Autodesk Inventor part; units mm, degrees
(part 2 of 3)
  circle A482 centre (-130.67, 0.7875) radius 0.851
  circle A483 centre (-28.5938, 38.8875) radius 1.994
  circle A484 centre (-33.6737, 38.8875) radius 0.851
  circle A485 centre (-23.5138, 38.8875) radius 0.851
  circle A486 centre (-19.0688, 19.8375) radius 1.994
  circle A487 centre (-24.1488, 19.8375) radius 0.851
  circle A488 centre (-13.9888, 19.8375) radius 0.851
  circle A489 centre (-14.3063, 0.7875) radius 1.994
  circle A490 centre (-19.3863, 0.7875) radius 0.851
  circle A491 centre (-9.2263, 0.7875) radius 0.851
  circle A492 centre (-4.7812, -18.2625) radius 1.994
  circle A493 centre (-9.8613, -18.2625) radius 0.851
  circle A494 centre (0.2988, -18.2625) radius 0.851
  circle A495 centre (-21.45, -37.3125) radius 1.994
  circle A496 centre (-26.53, -37.3125) radius 0.851
  circle A497 centre (-16.37, -37.3125) radius 0.851
  circle A498 centre (-71.488, -30.3275) radius 1.524
  circle A499 centre (28.588, -30.3275) radius 1.524
  circle A500 centre (-71.488, -45.5675) radius 1.994
  circle A501 centre (28.588, -45.5675) radius 1.994
  circle A502 centre (-9.5437, 38.8875) radius 1.994
  circle A503 centre (-14.6237, 38.8875) radius 0.851
  circle A504 centre (-4.4638, 38.8875) radius 0.851
  circle A505 centre (-0.0187, 19.8375) radius 1.994
  circle A506 centre (-5.0987, 19.8375) radius 0.851
  circle A507 centre (5.0613, 19.8375) radius 0.851
  circle A508 centre (4.7438, 0.7875) radius 1.994
  circle A509 centre (-0.3363, 0.7875) radius 0.851
  circle A510 centre (9.8238, 0.7875) radius 0.851
  circle A511 centre (14.2688, -18.2625) radius 1.994
  circle A512 centre (9.1888, -18.2625) radius 0.851
  circle A513 centre (19.3487, -18.2625) radius 0.851
  circle A514 centre (-130.9875, -18.2625) radius 1.994
  circle A515 centre (-136.0675, -18.2625) radius 0.851
  circle A516 centre (-125.9075, -18.2625) radius 0.851
  circle A517 centre (-142.9255, -11.2775) radius 1.524
  circle A518 centre (-119.0495, -11.2775) radius 1.524
  circle A519 centre (-142.9255, -26.5175) radius 1.994
  circle A520 centre (-119.0495, -26.5175) radius 1.994
  circle A521 centre (9.5063, 38.8875) radius 1.994
  circle A522 centre (4.4262, 38.8875) radius 0.851
  circle A523 centre (14.5862, 38.8875) radius 0.851
  circle A524 centre (19.0312, 19.8375) radius 1.994
  circle A525 centre (13.9513, 19.8375) radius 0.851
  circle A526 centre (24.1113, 19.8375) radius 0.851
  circle A527 centre (23.7937, 0.7875) radius 1.994
  circle A528 centre (18.7138, 0.7875) radius 0.851
  circle A529 centre (28.8738, 0.7875) radius 0.851
  circle A530 centre (33.3188, -18.2625) radius 1.994
  circle A531 centre (28.2388, -18.2625) radius 0.851
  circle A532 centre (38.3987, -18.2625) radius 0.851
  circle A533 centre (28.5562, 38.8875) radius 1.994
  circle A534 centre (23.4763, 38.8875) radius 0.851
  circle A535 centre (33.6362, 38.8875) radius 0.851
  circle A536 centre (38.0812, 19.8375) radius 1.994
  circle A537 centre (33.0012, 19.8375) radius 0.851
  circle A538 centre (43.1613, 19.8375) radius 0.851
  circle A539 centre (42.8438, 0.7875) radius 1.994
  circle A540 centre (37.7638, 0.7875) radius 0.851
  circle A541 centre (47.9237, 0.7875) radius 0.851
  circle A542 centre (52.3688, -18.2625) radius 1.994
  circle A543 centre (47.2888, -18.2625) radius 0.851
  circle A544 centre (57.4488, -18.2625) radius 0.851
  circle A545 centre (-140.5125, -37.3125) radius 1.994
  circle A546 centre (-145.5925, -37.3125) radius 0.851
  circle A547 centre (-135.4325, -37.3125) radius 0.851
  circle A548 centre (47.6063, 38.8875) radius 1.994
  circle A549 centre (42.5263, 38.8875) radius 0.851
  circle A550 centre (52.6863, 38.8875) radius 0.851
  circle A551 centre (57.1313, 19.8375) radius 1.994
  circle A552 centre (52.0513, 19.8375) radius 0.851
  circle A553 centre (62.2113, 19.8375) radius 0.851
  circle A554 centre (61.8937, 0.7875) radius 1.994
  circle A555 centre (56.8137, 0.7875) radius 0.851
  circle A556 centre (66.9737, 0.7875) radius 0.851
  circle A557 centre (71.4188, -18.2625) radius 1.994
  circle A558 centre (66.3388, -18.2625) radius 0.851
  circle A559 centre (76.4988, -18.2625) radius 0.851
  circle A560 centre (47.6063, -37.3125) radius 1.994
  circle A561 centre (42.5263, -37.3125) radius 0.851
  circle A562 centre (52.6863, -37.3125) radius 0.851
  circle A563 centre (66.6562, 38.8875) radius 1.994
  circle A564 centre (61.5763, 38.8875) radius 0.851
  circle A565 centre (71.7362, 38.8875) radius 0.851
  circle A566 centre (76.1813, 19.8375) radius 1.994
  circle A567 centre (71.1012, 19.8375) radius 0.851
  circle A568 centre (81.2613, 19.8375) radius 0.851
  circle A569 centre (80.9437, 0.7875) radius 1.994
  circle A570 centre (75.8638, 0.7875) radius 0.851
  circle A571 centre (86.0238, 0.7875) radius 0.851
  circle A572 centre (97.6125, -18.2625) radius 1.994
  circle A573 centre (92.5325, -18.2625) radius 0.851
  circle A574 centre (102.6925, -18.2625) radius 0.851
  circle A575 centre (-123.8438, 38.8875) radius 1.994
  circle A576 centre (-128.9238, 38.8875) radius 0.851
  circle A577 centre (-118.7638, 38.8875) radius 0.851
  circle A578 centre (66.6562, -37.3125) radius 1.994
  circle A579 centre (61.5763, -37.3125) radius 0.851
  circle A580 centre (71.7362, -37.3125) radius 0.851
  circle A581 centre (85.7062, 38.8875) radius 1.994
  circle A582 centre (80.6262, 38.8875) radius 0.851
  circle A583 centre (90.7863, 38.8875) radius 0.851
  circle A584 centre (95.2313, 19.8375) radius 1.994
  circle A585 centre (90.1513, 19.8375) radius 0.851
  circle A586 centre (100.3113, 19.8375) radius 0.851
  circle A587 centre (111.9, 0.7875) radius 1.994
  circle A588 centre (106.82, 0.7875) radius 0.851
  circle A589 centre (116.98, 0.7875) radius 0.851
  circle A590 centre (99.962, 7.7725) radius 1.524
  circle A591 centre (123.838, 7.7725) radius 1.524
  circle A592 centre (99.962, -7.4675) radius 1.994
  circle A593 centre (123.838, -7.4675) radius 1.994
  circle A594 centre (123.8063, -18.2625) radius 1.994
  circle A595 centre (118.7262, -18.2625) radius 0.851
  circle A596 centre (128.8862, -18.2625) radius 0.851
  circle A597 centre (85.7062, -37.3125) radius 1.994
  circle A598 centre (80.6262, -37.3125) radius 0.851
  circle A599 centre (90.7863, -37.3125) radius 0.851
  circle A600 centre (114.2813, 38.8875) radius 1.994
  circle A601 centre (109.2013, 38.8875) radius 0.851
  circle A602 centre (119.3613, 38.8875) radius 0.851
  circle A603 centre (102.3432, 45.8725) radius 1.524
  circle A604 centre (126.2193, 45.8725) radius 1.524
  circle A605 centre (102.3432, 30.6325) radius 1.994
  circle A606 centre (126.2193, 30.6325) radius 1.994
  circle A607 centre (119.0438, 19.8375) radius 1.994
  circle A608 centre (113.9638, 19.8375) radius 0.851
  circle A609 centre (124.1238, 19.8375) radius 0.851
  circle A610 centre (142.8562, 0.7875) radius 1.994
  circle A611 centre (137.7763, 0.7875) radius 0.851
  circle A612 centre (147.9363, 0.7875) radius 0.851
  circle A613 centre (142.8562, -18.2625) radius 1.994
  circle A614 centre (137.7763, -18.2625) radius 0.851
  circle A615 centre (147.9363, -18.2625) radius 0.851
  circle A616 centre (-114.3187, 19.8375) radius 1.994
  circle A617 centre (-119.3988, 19.8375) radius 0.851
  circle A618 centre (-109.2388, 19.8375) radius 0.851
  circle A619 centre (123.8063, -37.3125) radius 1.994
  circle A620 centre (118.7262, -37.3125) radius 0.851
  circle A621 centre (128.8862, -37.3125) radius 0.851
  circle A622 centre (142.8562, 38.8875) radius 1.994
  circle A623 centre (137.7763, 38.8875) radius 0.851
  circle A624 centre (147.9363, 38.8875) radius 0.851
  circle A625 centre (142.8562, 19.8375) radius 1.994
  circle A626 centre (137.7763, 19.8375) radius 0.851
  circle A627 centre (147.9363, 19.8375) radius 0.851
  circle A628 centre (104.7563, -37.3125) radius 1.994
  circle A629 centre (99.6762, -37.3125) radius 0.851
  circle A630 centre (109.8363, -37.3125) radius 0.851
  circle A631 centre (142.8562, -37.3125) radius 1.994
  circle A632 centre (137.7763, -37.3125) radius 0.851
  circle A633 centre (147.9363, -37.3125) radius 0.851
  circle A634 centre (-109.5563, 0.7875) radius 1.994
  circle A635 centre (-114.6363, 0.7875) radius 0.851
  circle A636 centre (-104.4763, 0.7875) radius 0.851
  circle A637 centre (-100.0312, -18.2625) radius 1.994
  circle A638 centre (-105.1112, -18.2625) radius 0.851
  circle A639 centre (-94.9513, -18.2625) radius 0.851
  line L281 (-145.2377, 58) -> (-145.2377, 70.7)
  line L282 (-153.25, 48.1608) -> (-159.6, 48.1608)
  line L283 (144.4828, -58) -> (144.4828, -70.7)
  line L284 (153.25, -45.7916) -> (159.6, -45.7916)
  line L285 (-159.6, 70.7) -> (159.6, 70.7)
  line L286 (159.6, 70.7) -> (159.6, -70.7)
  line L287 (159.6, -70.7) -> (-159.6, -70.7)
  line L288 (-159.6, -70.7) -> (-159.6, 70.7)
  line L289 (-149.6121, 31.8644) -> (-136.1755, 31.8644)
  line L290 (-135.8706, 32.1692) -> (-135.8706, 45.6058)
  line L291 (-136.1755, 45.9106) -> (-149.6121, 45.9106)
  line L292 (-149.9169, 45.6058) -> (-149.9169, 32.1692)
  line L293 (-149.9169, 31.8644) -> (-135.8706, 45.9106) construction
  line L294 (-135.8706, 31.8644) -> (-149.9169, 45.9106) construction
  arc A640 (-149.6121, 45.9106) -> (-149.9169, 45.6058) centre (-149.6121, 45.6058) ccw
  arc A641 (-135.8706, 45.6058) -> (-136.1755, 45.9106) centre (-136.1755, 45.6058) ccw
  arc A642 (-136.1755, 31.8644) -> (-135.8706, 32.1692) centre (-136.1755, 32.1692) ccw
  arc A643 (-149.9169, 32.1692) -> (-149.6121, 31.8644) centre (-149.6121, 32.1692) ccw
  line L295 (-130.562, 31.8644) -> (-117.1254, 31.8644)
  line L296 (-116.8206, 32.1692) -> (-116.8206, 45.6058)
  line L297 (-117.1254, 45.9106) -> (-130.562, 45.9106)
  line L298 (-130.8668, 45.6058) -> (-130.8668, 32.1692)
  line L299 (-130.8668, 31.8644) -> (-116.8206, 45.9106) construction
  line L300 (-116.8206, 31.8644) -> (-130.8668, 45.9106) construction
  arc A644 (-130.562, 45.9106) -> (-130.8668, 45.6058) centre (-130.562, 45.6058) ccw
  arc A645 (-116.8206, 45.6058) -> (-117.1254, 45.9106) centre (-117.1254, 45.6058) ccw
  arc A646 (-117.1254, 31.8644) -> (-116.8206, 32.1692) centre (-117.1254, 32.1692) ccw
  arc A647 (-130.8668, 32.1692) -> (-130.562, 31.8644) centre (-130.562, 32.1692) ccw
  line L301 (-111.5121, 31.8644) -> (-98.0754, 31.8644)
  line L302 (-97.7706, 32.1692) -> (-97.7706, 45.6058)
  line L303 (-98.0754, 45.9106) -> (-111.5121, 45.9106)
  line L304 (-111.8169, 45.6058) -> (-111.8169, 32.1692)
  line L305 (-111.8169, 31.8644) -> (-97.7706, 45.9106) construction
  line L306 (-97.7706, 31.8644) -> (-111.8169, 45.9106) construction
  arc A648 (-111.5121, 45.9106) -> (-111.8169, 45.6058) centre (-111.5121, 45.6058) ccw
  arc A649 (-97.7706, 45.6058) -> (-98.0754, 45.9106) centre (-98.0754, 45.6058) ccw
  arc A650 (-98.0754, 31.8644) -> (-97.7706, 32.1692) centre (-98.0754, 32.1692) ccw
  arc A651 (-111.8169, 32.1692) -> (-111.5121, 31.8644) centre (-111.512, 32.1692) ccw
  line L307 (-92.4621, 31.8644) -> (-79.0254, 31.8644)
  line L308 (-78.7206, 32.1692) -> (-78.7206, 45.6058)
  line L309 (-79.0254, 45.9106) -> (-92.4621, 45.9106)
  line L310 (-92.7669, 45.6058) -> (-92.7669, 32.1692)
  line L311 (-92.7669, 31.8644) -> (-78.7206, 45.9106) construction
  line L312 (-78.7206, 31.8644) -> (-92.7669, 45.9106) construction
  arc A652 (-92.4621, 45.9106) -> (-92.7669, 45.6058) centre (-92.4621, 45.6058) ccw
  arc A653 (-78.7206, 45.6058) -> (-79.0254, 45.9106) centre (-79.0255, 45.6058) ccw
  arc A654 (-79.0254, 31.8644) -> (-78.7206, 32.1692) centre (-79.0255, 32.1692) ccw
  arc A655 (-92.7669, 32.1692) -> (-92.4621, 31.8644) centre (-92.4621, 32.1692) ccw
  line L313 (-73.412, 31.8644) -> (-59.9754, 31.8644)
  line L314 (-59.6706, 32.1692) -> (-59.6706, 45.6058)
  line L315 (-59.9754, 45.9106) -> (-73.412, 45.9106)
  line L316 (-73.7168, 45.6058) -> (-73.7168, 32.1692)
  line L317 (-73.7168, 31.8644) -> (-59.6706, 45.9106) construction
  line L318 (-59.6706, 31.8644) -> (-73.7168, 45.9106) construction
  arc A656 (-73.412, 45.9106) -> (-73.7168, 45.6058) centre (-73.412, 45.6058) ccw
  arc A657 (-59.6706, 45.6058) -> (-59.9754, 45.9106) centre (-59.9754, 45.6058) ccw
  arc A658 (-59.9754, 31.8644) -> (-59.6706, 32.1692) centre (-59.9754, 32.1692) ccw
  arc A659 (-73.7168, 32.1692) -> (-73.412, 31.8644) centre (-73.412, 32.1692) ccw
  line L319 (-54.3621, 31.8644) -> (-40.9254, 31.8644)
  line L320 (-40.6206, 32.1692) -> (-40.6206, 45.6058)
  line L321 (-40.9254, 45.9106) -> (-54.3621, 45.9106)
  line L322 (-54.6668, 45.6058) -> (-54.6668, 32.1692)
  line L323 (-54.6668, 31.8644) -> (-40.6206, 45.9106) construction
  line L324 (-40.6206, 31.8644) -> (-54.6668, 45.9106) construction
  arc A660 (-54.3621, 45.9106) -> (-54.6668, 45.6058) centre (-54.3621, 45.6058) ccw
  arc A661 (-40.6206, 45.6058) -> (-40.9254, 45.9106) centre (-40.9254, 45.6058) ccw
  arc A662 (-40.9254, 31.8644) -> (-40.6206, 32.1692) centre (-40.9254, 32.1692) ccw
  arc A663 (-54.6668, 32.1692) -> (-54.3621, 31.8644) centre (-54.362, 32.1692) ccw
  line L325 (-35.312, 31.8644) -> (-21.8754, 31.8644)
  line L326 (-21.5706, 32.1692) -> (-21.5706, 45.6058)
  line L327 (-21.8754, 45.9106) -> (-35.312, 45.9106)
  line L328 (-35.6168, 45.6058) -> (-35.6168, 32.1692)
  line L329 (-35.6168, 31.8644) -> (-21.5706, 45.9106) construction
  line L330 (-21.5706, 31.8644) -> (-35.6168, 45.9106) construction
  arc A664 (-35.312, 45.9106) -> (-35.6168, 45.6058) centre (-35.312, 45.6058) ccw
  arc A665 (-21.5706, 45.6058) -> (-21.8754, 45.9106) centre (-21.8754, 45.6058) ccw
  arc A666 (-21.8754, 31.8644) -> (-21.5706, 32.1692) centre (-21.8754, 32.1692) ccw
  arc A667 (-35.6168, 32.1692) -> (-35.312, 31.8644) centre (-35.312, 32.1692) ccw
  line L331 (-16.262, 31.8644) -> (-2.8254, 31.8644)
  line L332 (-2.5206, 32.1692) -> (-2.5206, 45.6058)
  line L333 (-2.8254, 45.9106) -> (-16.262, 45.9106)
  line L334 (-16.5668, 45.6058) -> (-16.5668, 32.1692)
  line L335 (-16.5668, 31.8644) -> (-2.5206, 45.9106) construction
  line L336 (-2.5206, 31.8644) -> (-16.5668, 45.9106) construction
  arc A668 (-16.262, 45.9106) -> (-16.5668, 45.6058) centre (-16.262, 45.6058) ccw
  arc A669 (-2.5206, 45.6058) -> (-2.8254, 45.9106) centre (-2.8254, 45.6058) ccw
  arc A670 (-2.8254, 31.8644) -> (-2.5206, 32.1692) centre (-2.8254, 32.1692) ccw
  arc A671 (-16.5668, 32.1692) -> (-16.262, 31.8644) centre (-16.262, 32.1692) ccw
  line L337 (2.788, 31.8644) -> (16.2246, 31.8644)
  line L338 (16.5294, 32.1692) -> (16.5294, 45.6058)
  line L339 (16.2246, 45.9106) -> (2.788, 45.9106)
  line L340 (2.4832, 45.6058) -> (2.4832, 32.1692)
  line L341 (2.4832, 31.8644) -> (16.5294, 45.9106) construction
  line L342 (16.5294, 31.8644) -> (2.4832, 45.9106) construction
  arc A672 (2.788, 45.9106) -> (2.4832, 45.6058) centre (2.788, 45.6058) ccw
  arc A673 (16.5294, 45.6058) -> (16.2246, 45.9106) centre (16.2246, 45.6058) ccw
  arc A674 (16.2246, 31.8644) -> (16.5294, 32.1692) centre (16.2246, 32.1692) ccw
  arc A675 (2.4832, 32.1692) -> (2.788, 31.8644) centre (2.788, 32.1692) ccw
  line L343 (21.838, 31.8644) -> (35.2746, 31.8644)
  line L344 (35.5794, 32.1692) -> (35.5794, 45.6058)
  line L345 (35.2746, 45.9106) -> (21.838, 45.9106)
  line L346 (21.5332, 45.6058) -> (21.5332, 32.1692)
  line L347 (21.5332, 31.8644) -> (35.5794, 45.9106) construction
  line L348 (35.5794, 31.8644) -> (21.5332, 45.9106) construction
  arc A676 (21.838, 45.9106) -> (21.5332, 45.6058) centre (21.838, 45.6058) ccw
  arc A677 (35.5794, 45.6058) -> (35.2746, 45.9106) centre (35.2746, 45.6058) ccw
  arc A678 (35.2746, 31.8644) -> (35.5794, 32.1692) centre (35.2746, 32.1692) ccw
  arc A679 (21.5332, 32.1692) -> (21.838, 31.8644) centre (21.838, 32.1692) ccw
  line L349 (40.888, 31.8644) -> (54.3246, 31.8644)
  line L350 (54.6294, 32.1692) -> (54.6294, 45.6058)
  line L351 (54.3246, 45.9106) -> (40.888, 45.9106)
  line L352 (40.5832, 45.6058) -> (40.5832, 32.1692)
  line L353 (40.5832, 31.8644) -> (54.6294, 45.9106) construction
  line L354 (54.6294, 31.8644) -> (40.5832, 45.9106) construction
  arc A680 (40.888, 45.9106) -> (40.5832, 45.6058) centre (40.888, 45.6058) ccw
  arc A681 (54.6294, 45.6058) -> (54.3246, 45.9106) centre (54.3246, 45.6058) ccw
  arc A682 (54.3246, 31.8644) -> (54.6294, 32.1692) centre (54.3246, 32.1692) ccw
  arc A683 (40.5832, 32.1692) -> (40.888, 31.8644) centre (40.888, 32.1692) ccw
  line L355 (59.938, 31.8644) -> (73.3746, 31.8644)
  line L356 (73.6794, 32.1692) -> (73.6794, 45.6058)
  line L357 (73.3746, 45.9106) -> (59.938, 45.9106)
  line L358 (59.6332, 45.6058) -> (59.6332, 32.1692)
  line L359 (59.6332, 31.8644) -> (73.6794, 45.9106) construction
  line L360 (73.6794, 31.8644) -> (59.6332, 45.9106) construction
  arc A684 (59.938, 45.9106) -> (59.6332, 45.6058) centre (59.938, 45.6058) ccw
  arc A685 (73.6794, 45.6058) -> (73.3746, 45.9106) centre (73.3746, 45.6058) ccw
  arc A686 (73.3746, 31.8644) -> (73.6794, 32.1692) centre (73.3746, 32.1692) ccw
  arc A687 (59.6332, 32.1692) -> (59.938, 31.8644) centre (59.938, 32.1692) ccw
  line L361 (78.988, 31.8644) -> (92.4246, 31.8644)
  line L362 (92.7294, 32.1692) -> (92.7294, 45.6058)
  line L363 (92.4246, 45.9106) -> (78.988, 45.9106)
  line L364 (78.6832, 45.6058) -> (78.6832, 32.1692)
  line L365 (78.6832, 31.8644) -> (92.7294, 45.9106) construction
  line L366 (92.7294, 31.8644) -> (78.6832, 45.9106) construction
  arc A688 (78.988, 45.9106) -> (78.6832, 45.6058) centre (78.988, 45.6058) ccw
  arc A689 (92.7294, 45.6058) -> (92.4246, 45.9106) centre (92.4246, 45.6058) ccw
  arc A690 (92.4246, 31.8644) -> (92.7294, 32.1692) centre (92.4246, 32.1692) ccw
  arc A691 (78.6832, 32.1692) -> (78.988, 31.8644) centre (78.988, 32.1692) ccw
  line L367 (136.1379, 31.8644) -> (149.5746, 31.8644)
  line L368 (149.8794, 32.1692) -> (149.8794, 45.6058)
  line L369 (149.5746, 45.9106) -> (136.1379, 45.9106)
  line L370 (135.8332, 45.6058) -> (135.8332, 32.1692)
  line L371 (135.8332, 31.8644) -> (149.8794, 45.9106) construction
  line L372 (149.8794, 31.8644) -> (135.8332, 45.9106) construction
  arc A692 (136.1379, 45.9106) -> (135.8332, 45.6058) centre (136.1379, 45.6058) ccw
  arc A693 (149.8794, 45.6058) -> (149.5746, 45.9106) centre (149.5746, 45.6058) ccw
  arc A694 (149.5746, 31.8644) -> (149.8794, 32.1692) centre (149.5746, 32.1692) ccw
  arc A695 (135.8332, 32.1692) -> (136.1379, 31.8644) centre (136.138, 32.1692) ccw
  line L373 (-121.037, 12.8144) -> (-107.6004, 12.8144)
  line L374 (-107.2956, 13.1192) -> (-107.2956, 26.5558)
  line L375 (-107.6004, 26.8606) -> (-121.037, 26.8606)
  line L376 (-121.3418, 26.5558) -> (-121.3418, 13.1192)
  line L377 (-121.3418, 12.8144) -> (-107.2956, 26.8606) construction
  line L378 (-107.2956, 12.8144) -> (-121.3418, 26.8606) construction
  arc A696 (-121.037, 26.8606) -> (-121.3418, 26.5558) centre (-121.037, 26.5558) ccw
  arc A697 (-107.2956, 26.5558) -> (-107.6004, 26.8606) centre (-107.6004, 26.5558) ccw
  arc A698 (-107.6004, 12.8144) -> (-107.2956, 13.1192) centre (-107.6004, 13.1192) ccw
  arc A699 (-121.3418, 13.1192) -> (-121.037, 12.8144) centre (-121.037, 13.1192) ccw
  line L379 (-101.9871, 12.8144) -> (-88.5504, 12.8144)
  line L380 (-88.2456, 13.1192) -> (-88.2456, 26.5558)
  line L381 (-88.5504, 26.8606) -> (-101.9871, 26.8606)
  line L382 (-102.2918, 26.5558) -> (-102.2918, 13.1192)
  line L383 (-102.2918, 12.8144) -> (-88.2456, 26.8606) construction
  line L384 (-88.2456, 12.8144) -> (-102.2918, 26.8606) construction
  arc A700 (-101.9871, 26.8606) -> (-102.2918, 26.5558) centre (-101.9871, 26.5558) ccw
  arc A701 (-88.2456, 26.5558) -> (-88.5504, 26.8606) centre (-88.5504, 26.5558) ccw
  arc A702 (-88.5504, 12.8144) -> (-88.2456, 13.1192) centre (-88.5504, 13.1192) ccw
  arc A703 (-102.2918, 13.1192) -> (-101.9871, 12.8144) centre (-101.987, 13.1192) ccw
  line L385 (-82.937, 12.8144) -> (-69.5004, 12.8144)
  line L386 (-69.1956, 13.1192) -> (-69.1956, 26.5558)
  line L387 (-69.5004, 26.8606) -> (-82.937, 26.8606)
  line L388 (-83.2418, 26.5558) -> (-83.2418, 13.1192)
  line L389 (-83.2418, 12.8144) -> (-69.1956, 26.8606) construction
  line L390 (-69.1956, 12.8144) -> (-83.2418, 26.8606) construction
  arc A704 (-82.937, 26.8606) -> (-83.2418, 26.5558) centre (-82.937, 26.5558) ccw
  arc A705 (-69.1956, 26.5558) -> (-69.5004, 26.8606) centre (-69.5005, 26.5558) ccw
  arc A706 (-69.5004, 12.8144) -> (-69.1956, 13.1192) centre (-69.5005, 13.1192) ccw
  arc A707 (-83.2418, 13.1192) -> (-82.937, 12.8144) centre (-82.937, 13.1192) ccw
  line L391 (-63.887, 12.8144) -> (-50.4504, 12.8144)
  line L392 (-50.1456, 13.1192) -> (-50.1456, 26.5558)
  line L393 (-50.4504, 26.8606) -> (-63.887, 26.8606)
  line L394 (-64.1918, 26.5558) -> (-64.1918, 13.1192)
  line L395 (-64.1918, 12.8144) -> (-50.1456, 26.8606) construction
  line L396 (-50.1456, 12.8144) -> (-64.1918, 26.8606) construction
  arc A708 (-63.887, 26.8606) -> (-64.1918, 26.5558) centre (-63.887, 26.5558) ccw
  arc A709 (-50.1456, 26.5558) -> (-50.4504, 26.8606) centre (-50.4504, 26.5558) ccw
  arc A710 (-50.4504, 12.8144) -> (-50.1456, 13.1192) centre (-50.4504, 13.1192) ccw
  arc A711 (-64.1918, 13.1192) -> (-63.887, 12.8144) centre (-63.887, 13.1192) ccw
  line L397 (-44.837, 12.8144) -> (-31.4004, 12.8144)
  line L398 (-31.0956, 13.1192) -> (-31.0956, 26.5558)
  line L399 (-31.4004, 26.8606) -> (-44.837, 26.8606)
  line L400 (-45.1418, 26.5558) -> (-45.1418, 13.1192)
  line L401 (-45.1418, 12.8144) -> (-31.0956, 26.8606) construction
  line L402 (-31.0956, 12.8144) -> (-45.1418, 26.8606) construction
  arc A712 (-44.837, 26.8606) -> (-45.1418, 26.5558) centre (-44.837, 26.5558) ccw
  arc A713 (-31.0956, 26.5558) -> (-31.4004, 26.8606) centre (-31.4004, 26.5558) ccw
  arc A714 (-31.4004, 12.8144) -> (-31.0956, 13.1192) centre (-31.4004, 13.1192) ccw
  arc A715 (-45.1418, 13.1192) -> (-44.837, 12.8144) centre (-44.837, 13.1192) ccw
  line L403 (-25.787, 12.8144) -> (-12.3504, 12.8144)
  line L404 (-12.0456, 13.1192) -> (-12.0456, 26.5558)
  line L405 (-12.3504, 26.8606) -> (-25.787, 26.8606)
  line L406 (-26.0918, 26.5558) -> (-26.0918, 13.1192)
  line L407 (-26.0918, 12.8144) -> (-12.0456, 26.8606) construction
  line L408 (-12.0456, 12.8144) -> (-26.0918, 26.8606) construction
  arc A716 (-25.787, 26.8606) -> (-26.0918, 26.5558) centre (-25.787, 26.5558) ccw
  arc A717 (-12.0456, 26.5558) -> (-12.3504, 26.8606) centre (-12.3504, 26.5558) ccw
  arc A718 (-12.3504, 12.8144) -> (-12.0456, 13.1192) centre (-12.3504, 13.1192) ccw
  arc A719 (-26.0918, 13.1192) -> (-25.787, 12.8144) centre (-25.787, 13.1192) ccw
  line L409 (-6.737, 12.8144) -> (6.6996, 12.8144)
  line L410 (7.0044, 13.1192) -> (7.0044, 26.5558)
  line L411 (6.6996, 26.8606) -> (-6.737, 26.8606)
  line L412 (-7.0418, 26.5558) -> (-7.0418, 13.1192)
  line L413 (-7.0418, 12.8144) -> (7.0044, 26.8606) construction
  line L414 (7.0044, 12.8144) -> (-7.0418, 26.8606) construction
  arc A720 (-6.737, 26.8606) -> (-7.0418, 26.5558) centre (-6.737, 26.5558) ccw
  arc A721 (7.0044, 26.5558) -> (6.6996, 26.8606) centre (6.6996, 26.5558) ccw
  arc A722 (6.6996, 12.8144) -> (7.0044, 13.1192) centre (6.6996, 13.1192) ccw
  arc A723 (-7.0418, 13.1192) -> (-6.737, 12.8144) centre (-6.737, 13.1192) ccw
  line L415 (12.313, 12.8144) -> (25.7496, 12.8144)
  line L416 (26.0544, 13.1192) -> (26.0544, 26.5558)
  line L417 (25.7496, 26.8606) -> (12.313, 26.8606)
  line L418 (12.0082, 26.5558) -> (12.0082, 13.1192)
  line L419 (12.0082, 12.8144) -> (26.0544, 26.8606) construction
  line L420 (26.0544, 12.8144) -> (12.0082, 26.8606) construction
  arc A724 (12.313, 26.8606) -> (12.0082, 26.5558) centre (12.313, 26.5558) ccw
  arc A725 (26.0544, 26.5558) -> (25.7496, 26.8606) centre (25.7496, 26.5558) ccw
  arc A726 (25.7496, 12.8144) -> (26.0544, 13.1192) centre (25.7496, 13.1192) ccw
  arc A727 (12.0082, 13.1192) -> (12.313, 12.8144) centre (12.313, 13.1192) ccw
  line L421 (31.363, 12.8144) -> (44.7996, 12.8144)
  line L422 (45.1044, 13.1192) -> (45.1044, 26.5558)
  line L423 (44.7996, 26.8606) -> (31.363, 26.8606)
  line L424 (31.0582, 26.5558) -> (31.0582, 13.1192)
  line L425 (31.0582, 12.8144) -> (45.1044, 26.8606) construction
  line L426 (45.1044, 12.8144) -> (31.0582, 26.8606) construction
  arc A728 (31.363, 26.8606) -> (31.0582, 26.5558) centre (31.363, 26.5558) ccw
  arc A729 (45.1044, 26.5558) -> (44.7996, 26.8606) centre (44.7996, 26.5558) ccw
  arc A730 (44.7996, 12.8144) -> (45.1044, 13.1192) centre (44.7996, 13.1192) ccw
  arc A731 (31.0582, 13.1192) -> (31.363, 12.8144) centre (31.363, 13.1192) ccw
  line L427 (50.413, 12.8144) -> (63.8496, 12.8144)
  line L428 (64.1544, 13.1192) -> (64.1544, 26.5558)
  line L429 (63.8496, 26.8606) -> (50.413, 26.8606)
  line L430 (50.1082, 26.5558) -> (50.1082, 13.1192)
  line L431 (50.1082, 12.8144) -> (64.1544, 26.8606) construction
  line L432 (64.1544, 12.8144) -> (50.1082, 26.8606) construction
  arc A732 (50.413, 26.8606) -> (50.1082, 26.5558) centre (50.413, 26.5558) ccw
  arc A733 (64.1544, 26.5558) -> (63.8496, 26.8606) centre (63.8496, 26.5558) ccw
  arc A734 (63.8496, 12.8144) -> (64.1544, 13.1192) centre (63.8496, 13.1192) ccw
  arc A735 (50.1082, 13.1192) -> (50.413, 12.8144) centre (50.413, 13.1192) ccw
  line L433 (69.463, 12.8144) -> (82.8996, 12.8144)
  line L434 (83.2044, 13.1192) -> (83.2044, 26.5558)
  line L435 (82.8996, 26.8606) -> (69.463, 26.8606)
  line L436 (69.1582, 26.5558) -> (69.1582, 13.1192)
  line L437 (69.1582, 12.8144) -> (83.2044, 26.8606) construction
  line L438 (83.2044, 12.8144) -> (69.1582, 26.8606) construction
  arc A736 (69.463, 26.8606) -> (69.1582, 26.5558) centre (69.463, 26.5558) ccw
  arc A737 (83.2044, 26.5558) -> (82.8996, 26.8606) centre (82.8996, 26.5558) ccw
  arc A738 (82.8996, 12.8144) -> (83.2044, 13.1192) centre (82.8996, 13.1192) ccw
  arc A739 (69.1582, 13.1192) -> (69.463, 12.8144) centre (69.463, 13.1192) ccw
  line L439 (88.513, 12.8144) -> (101.9496, 12.8144)
  line L440 (102.2544, 13.1192) -> (102.2544, 26.5558)
  line L441 (101.9496, 26.8606) -> (88.513, 26.8606)
  line L442 (88.2082, 26.5558) -> (88.2082, 13.1192)
  line L443 (88.2082, 12.8144) -> (102.2544, 26.8606) construction
  line L444 (102.2544, 12.8144) -> (88.2082, 26.8606) construction
  arc A740 (88.513, 26.8606) -> (88.2082, 26.5558) centre (88.513, 26.5558) ccw
  arc A741 (102.2544, 26.5558) -> (101.9496, 26.8606) centre (101.9496, 26.5558) ccw
  arc A742 (101.9496, 12.8144) -> (102.2544, 13.1192) centre (101.9496, 13.1192) ccw
  arc A743 (88.2082, 13.1192) -> (88.513, 12.8144) centre (88.513, 13.1192) ccw
  line L445 (136.1379, 12.8144) -> (149.5746, 12.8144)
  line L446 (149.8794, 13.1192) -> (149.8794, 26.5558)
  line L447 (149.5746, 26.8606) -> (136.1379, 26.8606)
  line L448 (135.8332, 26.5558) -> (135.8332, 13.1192)
  line L449 (135.8332, 12.8144) -> (149.8794, 26.8606) construction
  line L450 (149.8794, 12.8144) -> (135.8332, 26.8606) construction
  arc A744 (136.1379, 26.8606) -> (135.8332, 26.5558) centre (136.1379, 26.5558) ccw
  arc A745 (149.8794, 26.5558) -> (149.5746, 26.8606) centre (149.5746, 26.5558) ccw
  arc A746 (149.5746, 12.8144) -> (149.8794, 13.1192) centre (149.5746, 13.1192) ccw
  arc A747 (135.8332, 13.1192) -> (136.1379, 12.8144) centre (136.138, 13.1192) ccw
  line L451 (-116.2746, -6.2356) -> (-102.8379, -6.2356)
  line L452 (-102.5331, -5.9308) -> (-102.5331, 7.5058)
  line L453 (-102.8379, 7.8106) -> (-116.2746, 7.8106)
  line L454 (-116.5794, 7.5058) -> (-116.5794, -5.9308)
  line L455 (-116.5794, -6.2356) -> (-102.5331, 7.8106) construction
  line L456 (-102.5331, -6.2356) -> (-116.5794, 7.8106) construction
  arc A748 (-116.2746, 7.8106) -> (-116.5794, 7.5058) centre (-116.2746, 7.5058) ccw
  arc A749 (-102.5331, 7.5058) -> (-102.8379, 7.8106) centre (-102.8379, 7.5058) ccw
  arc A750 (-102.8379, -6.2356) -> (-102.5331, -5.9308) centre (-102.8379, -5.9308) ccw
  arc A751 (-116.5794, -5.9308) -> (-116.2746, -6.2356) centre (-116.2745, -5.9308) ccw
  line L457 (-97.2245, -6.2356) -> (-83.7879, -6.2356)
  line L458 (-83.4831, -5.9308) -> (-83.4831, 7.5058)
  line L459 (-83.7879, 7.8106) -> (-97.2245, 7.8106)
  line L460 (-97.5293, 7.5058) -> (-97.5293, -5.9308)
  line L461 (-97.5293, -6.2356) -> (-83.4831, 7.8106) construction
  line L462 (-83.4831, -6.2356) -> (-97.5293, 7.8106) construction
  arc A752 (-97.2245, 7.8106) -> (-97.5293, 7.5058) centre (-97.2245, 7.5058) ccw
  arc A753 (-83.4831, 7.5058) -> (-83.7879, 7.8106) centre (-83.7879, 7.5058) ccw
  arc A754 (-83.7879, -6.2356) -> (-83.4831, -5.9308) centre (-83.7879, -5.9308) ccw
  arc A755 (-97.5293, -5.9308) -> (-97.2245, -6.2356) centre (-97.2245, -5.9308) ccw
  line L463 (-78.1745, -6.2356) -> (-64.7379, -6.2356)
  line L464 (-64.4331, -5.9308) -> (-64.4331, 7.5058)
  line L465 (-64.7379, 7.8106) -> (-78.1745, 7.8106)
  line L466 (-78.4793, 7.5058) -> (-78.4793, -5.9308)
  line L467 (-78.4793, -6.2356) -> (-64.4331, 7.8106) construction
  line L468 (-64.4331, -6.2356) -> (-78.4793, 7.8106) construction
  arc A756 (-78.1745, 7.8106) -> (-78.4793, 7.5058) centre (-78.1745, 7.5058) ccw
  arc A757 (-64.4331, 7.5058) -> (-64.7379, 7.8106) centre (-64.7379, 7.5058) ccw
  arc A758 (-64.7379, -6.2356) -> (-64.4331, -5.9308) centre (-64.7379, -5.9308) ccw
  arc A759 (-78.4793, -5.9308) -> (-78.1745, -6.2356) centre (-78.1745, -5.9308) ccw
  line L469 (-59.1245, -6.2356) -> (-45.6879, -6.2356)
  line L470 (-45.3831, -5.9308) -> (-45.3831, 7.5058)
  line L471 (-45.6879, 7.8106) -> (-59.1245, 7.8106)
  line L472 (-59.4293, 7.5058) -> (-59.4293, -5.9308)
  line L473 (-59.4293, -6.2356) -> (-45.3831, 7.8106) construction
  line L474 (-45.3831, -6.2356) -> (-59.4293, 7.8106) construction
  arc A760 (-59.1245, 7.8106) -> (-59.4293, 7.5058) centre (-59.1245, 7.5058) ccw
  arc A761 (-45.3831, 7.5058) -> (-45.6879, 7.8106) centre (-45.6879, 7.5058) ccw
  arc A762 (-45.6879, -6.2356) -> (-45.3831, -5.9308) centre (-45.6879, -5.9308) ccw
  arc A763 (-59.4293, -5.9308) -> (-59.1245, -6.2356) centre (-59.1245, -5.9308) ccw
  line L475 (-40.0745, -6.2356) -> (-26.6379, -6.2356)
  line L476 (-26.3331, -5.9308) -> (-26.3331, 7.5058)
  line L477 (-26.6379, 7.8106) -> (-40.0745, 7.8106)
  line L478 (-40.3793, 7.5058) -> (-40.3793, -5.9308)
  line L479 (-40.3793, -6.2356) -> (-26.3331, 7.8106) construction
  line L480 (-26.3331, -6.2356) -> (-40.3793, 7.8106) construction
  arc A764 (-40.0745, 7.8106) -> (-40.3793, 7.5058) centre (-40.0745, 7.5058) ccw
  arc A765 (-26.3331, 7.5058) -> (-26.6379, 7.8106) centre (-26.6379, 7.5058) ccw
  arc A766 (-26.6379, -6.2356) -> (-26.3331, -5.9308) centre (-26.6379, -5.9308) ccw
  arc A767 (-40.3793, -5.9308) -> (-40.0745, -6.2356) centre (-40.0745, -5.9308) ccw
  line L481 (-21.0245, -6.2356) -> (-7.5879, -6.2356)
  line L482 (-7.2831, -5.9308) -> (-7.2831, 7.5058)
  line L483 (-7.5879, 7.8106) -> (-21.0245, 7.8106)
  line L484 (-21.3293, 7.5058) -> (-21.3293, -5.9308)
  line L485 (-21.3293, -6.2356) -> (-7.2831, 7.8106) construction
  line L486 (-7.2831, -6.2356) -> (-21.3293, 7.8106) construction
  arc A768 (-21.0245, 7.8106) -> (-21.3293, 7.5058) centre (-21.0245, 7.5058) ccw
  arc A769 (-7.2831, 7.5058) -> (-7.5879, 7.8106) centre (-7.5879, 7.5058) ccw
  arc A770 (-7.5879, -6.2356) -> (-7.2831, -5.9308) centre (-7.5879, -5.9308) ccw
  arc A771 (-21.3293, -5.9308) -> (-21.0245, -6.2356) centre (-21.0245, -5.9308) ccw
  line L487 (-1.9745, -6.2356) -> (11.4621, -6.2356)
  line L488 (11.7669, -5.9308) -> (11.7669, 7.5058)
  line L489 (11.4621, 7.8106) -> (-1.9745, 7.8106)
  line L490 (-2.2793, 7.5058) -> (-2.2793, -5.9308)
  line L491 (-2.2793, -6.2356) -> (11.7669, 7.8106) construction
  line L492 (11.7669, -6.2356) -> (-2.2793, 7.8106) construction
  arc A772 (-1.9745, 7.8106) -> (-2.2793, 7.5058) centre (-1.9745, 7.5058) ccw
  arc A773 (11.7669, 7.5058) -> (11.4621, 7.8106) centre (11.4621, 7.5058) ccw
  arc A774 (11.4621, -6.2356) -> (11.7669, -5.9308) centre (11.4621, -5.9308) ccw
  arc A775 (-2.2793, -5.9308) -> (-1.9745, -6.2356) centre (-1.9745, -5.9308) ccw
  line L493 (17.0755, -6.2356) -> (30.5121, -6.2356)
  line L494 (30.8169, -5.9308) -> (30.8169, 7.5058)
  line L495 (30.5121, 7.8106) -> (17.0755, 7.8106)
  line L496 (16.7707, 7.5058) -> (16.7707, -5.9308)
  line L497 (16.7707, -6.2356) -> (30.8169, 7.8106) construction
  line L498 (30.8169, -6.2356) -> (16.7707, 7.8106) construction
  arc A776 (17.0755, 7.8106) -> (16.7707, 7.5058) centre (17.0755, 7.5058) ccw
  arc A777 (30.8169, 7.5058) -> (30.5121, 7.8106) centre (30.5121, 7.5058) ccw
  arc A778 (30.5121, -6.2356) -> (30.8169, -5.9308) centre (30.5121, -5.9308) ccw
  arc A779 (16.7707, -5.9308) -> (17.0755, -6.2356) centre (17.0755, -5.9308) ccw
  line L499 (36.1255, -6.2356) -> (49.5621, -6.2356)
  line L500 (49.8669, -5.9308) -> (49.8669, 7.5058)
  line L501 (49.5621, 7.8106) -> (36.1255, 7.8106)
  line L502 (35.8207, 7.5058) -> (35.8207, -5.9308)
  line L503 (35.8207, -6.2356) -> (49.8669, 7.8106) construction
  line L504 (49.8669, -6.2356) -> (35.8207, 7.8106) construction
  arc A780 (36.1255, 7.8106) -> (35.8207, 7.5058) centre (36.1255, 7.5058) ccw
  arc A781 (49.8669, 7.5058) -> (49.5621, 7.8106) centre (49.5621, 7.5058) ccw
  arc A782 (49.5621, -6.2356) -> (49.8669, -5.9308) centre (49.5621, -5.9308) ccw
  arc A783 (35.8207, -5.9308) -> (36.1255, -6.2356) centre (36.1255, -5.9308) ccw
  line L505 (55.1755, -6.2356) -> (68.6121, -6.2356)
  line L506 (68.9169, -5.9308) -> (68.9169, 7.5058)
  line L507 (68.6121, 7.8106) -> (55.1755, 7.8106)
  line L508 (54.8707, 7.5058) -> (54.8707, -5.9308)
  line L509 (54.8707, -6.2356) -> (68.9169, 7.8106) construction
  line L510 (68.9169, -6.2356) -> (54.8707, 7.8106) construction
  arc A784 (55.1755, 7.8106) -> (54.8707, 7.5058) centre (55.1755, 7.5058) ccw
  arc A785 (68.9169, 7.5058) -> (68.6121, 7.8106) centre (68.6121, 7.5058) ccw
  arc A786 (68.6121, -6.2356) -> (68.9169, -5.9308) centre (68.6121, -5.9308) ccw
  arc A787 (54.8707, -5.9308) -> (55.1755, -6.2356) centre (55.1755, -5.9308) ccw
  line L511 (74.2255, -6.2356) -> (87.6621, -6.2356)
  line L512 (87.9669, -5.9308) -> (87.9669, 7.5058)
  line L513 (87.6621, 7.8106) -> (74.2255, 7.8106)
  line L514 (73.9207, 7.5058) -> (73.9207, -5.9308)
  line L515 (73.9207, -6.2356) -> (87.9669, 7.8106) construction
  line L516 (87.9669, -6.2356) -> (73.9207, 7.8106) construction
  arc A788 (74.2255, 7.8106) -> (73.9207, 7.5058) centre (74.2255, 7.5058) ccw
  arc A789 (87.9669, 7.5058) -> (87.6621, 7.8106) centre (87.6621, 7.5058) ccw
  arc A790 (87.6621, -6.2356) -> (87.9669, -5.9308) centre (87.6621, -5.9308) ccw
  arc A791 (73.9207, -5.9308) -> (74.2255, -6.2356) centre (74.2255, -5.9308) ccw
  line L517 (136.1379, -6.2356) -> (149.5746, -6.2356)
  line L518 (149.8794, -5.9308) -> (149.8794, 7.5058)
  line L519 (149.5746, 7.8106) -> (136.1379, 7.8106)
  line L520 (135.8332, 7.5058) -> (135.8332, -5.9308)
  line L521 (135.8332, -6.2356) -> (149.8794, 7.8106) construction
  line L522 (149.8794, -6.2356) -> (135.8332, 7.8106) construction
  arc A792 (136.1379, 7.8106) -> (135.8332, 7.5058) centre (136.1379, 7.5058) ccw
  arc A793 (149.8794, 7.5058) -> (149.5746, 7.8106) centre (149.5746, 7.5058) ccw
  arc A794 (149.5746, -6.2356) -> (149.8794, -5.9308) centre (149.5746, -5.9308) ccw
  arc A795 (135.8332, -5.9308) -> (136.1379, -6.2356) centre (136.138, -5.9308) ccw
  line L523 (-106.7495, -25.2856) -> (-93.3129, -25.2856)
  line L524 (-93.0081, -24.9808) -> (-93.0081, -11.5442)
  line L525 (-93.3129, -11.2394) -> (-106.7495, -11.2394)
  line L526 (-107.0543, -11.5442) -> (-107.0543, -24.9808)
  line L527 (-107.0543, -25.2856) -> (-93.0081, -11.2394) construction
  line L528 (-93.0081, -25.2856) -> (-107.0543, -11.2394) construction
  arc A796 (-106.7495, -11.2394) -> (-107.0543, -11.5442) centre (-106.7495, -11.5442) ccw
  arc A797 (-93.0081, -11.5442) -> (-93.3129, -11.2394) centre (-93.3129, -11.5442) ccw
  arc A798 (-93.3129, -25.2856) -> (-93.0081, -24.9808) centre (-93.3129, -24.9808) ccw
  arc A799 (-107.0543, -24.9808) -> (-106.7495, -25.2856) centre (-106.7495, -24.9808) ccw
  line L529 (-87.6995, -25.2856) -> (-74.2629, -25.2856)
  line L530 (-73.9581, -24.9808) -> (-73.9581, -11.5442)
  line L531 (-74.2629, -11.2394) -> (-87.6995, -11.2394)
  line L532 (-88.0044, -11.5442) -> (-88.0044, -24.9808)
  line L533 (-88.0044, -25.2856) -> (-73.9581, -11.2394) construction
  line L534 (-73.9581, -25.2856) -> (-88.0044, -11.2394) construction
  arc A800 (-87.6995, -11.2394) -> (-88.0044, -11.5442) centre (-87.6995, -11.5442) ccw
  arc A801 (-73.9581, -11.5442) -> (-74.2629, -11.2394) centre (-74.2629, -11.5442) ccw
  arc A802 (-74.2629, -25.2856) -> (-73.9581, -24.9808) centre (-74.2629, -24.9808) ccw
  arc A803 (-88.0044, -24.9808) -> (-87.6995, -25.2856) centre (-87.6995, -24.9808) ccw
  line L535 (-68.7073, -25.2278) -> (-55.2707, -25.2278)
  line L536 (-54.9659, -24.923) -> (-54.9659, -11.4864)
  line L537 (-55.2707, -11.1816) -> (-68.7073, -11.1816)
  line L538 (-69.0121, -11.4864) -> (-69.0121, -24.923)
  line L539 (-69.0121, -25.2278) -> (-54.9659, -11.1816) construction
  line L540 (-54.9659, -25.2278) -> (-69.0121, -11.1816) construction
  arc A804 (-68.7073, -11.1816) -> (-69.0121, -11.4864) centre (-68.7073, -11.4864) ccw
  arc A805 (-54.9659, -11.4864) -> (-55.2707, -11.1816) centre (-55.2707, -11.4864) ccw
  arc A806 (-55.2707, -25.2278) -> (-54.9659, -24.923) centre (-55.2707, -24.923) ccw
  arc A807 (-69.0121, -24.923) -> (-68.7073, -25.2278) centre (-68.7073, -24.923) ccw
  line L541 (-49.5995, -25.2856) -> (-36.1629, -25.2856)
  line L542 (-35.8581, -24.9808) -> (-35.8581, -11.5442)
  line L543 (-36.1629, -11.2394) -> (-49.5995, -11.2394)
  line L544 (-49.9043, -11.5442) -> (-49.9043, -24.9808)
  line L545 (-49.9043, -25.2856) -> (-35.8581, -11.2394) construction
  line L546 (-35.8581, -25.2856) -> (-49.9043, -11.2394) construction
  arc A808 (-49.5995, -11.2394) -> (-49.9043, -11.5442) centre (-49.5995, -11.5442) ccw
  arc A809 (-35.8581, -11.5442) -> (-36.1629, -11.2394) centre (-36.1629, -11.5442) ccw
  arc A810 (-36.1629, -25.2856) -> (-35.8581, -24.9808) centre (-36.1629, -24.9808) ccw
  arc A811 (-49.9043, -24.9808) -> (-49.5995, -25.2856) centre (-49.5995, -24.9808) ccw
  line L547 (-30.5495, -25.2856) -> (-17.1129, -25.2856)
  line L548 (-16.8081, -24.9808) -> (-16.8081, -11.5442)
  line L549 (-17.1129, -11.2394) -> (-30.5495, -11.2394)
  line L550 (-30.8543, -11.5442) -> (-30.8543, -24.9808)
  line L551 (-30.8543, -25.2856) -> (-16.8081, -11.2394) construction
  line L552 (-16.8081, -25.2856) -> (-30.8543, -11.2394) construction
  arc A812 (-30.5495, -11.2394) -> (-30.8543, -11.5442) centre (-30.5495, -11.5442) ccw
  arc A813 (-16.8081, -11.5442) -> (-17.1129, -11.2394) centre (-17.1129, -11.5442) ccw
  arc A814 (-17.1129, -25.2856) -> (-16.8081, -24.9808) centre (-17.1129, -24.9808) ccw
  arc A815 (-30.8543, -24.9808) -> (-30.5495, -25.2856) centre (-30.5495, -24.9808) ccw
  line L553 (-11.4995, -25.2856) -> (1.9371, -25.2856)
  line L554 (2.2419, -24.9808) -> (2.2419, -11.5442)
  line L555 (1.9371, -11.2394) -> (-11.4995, -11.2394)
  line L556 (-11.8043, -11.5442) -> (-11.8043, -24.9808)
  line L557 (-11.8043, -25.2856) -> (2.2419, -11.2394) construction
  line L558 (2.2419, -25.2856) -> (-11.8043, -11.2394) construction
  arc A816 (-11.4995, -11.2394) -> (-11.8043, -11.5442) centre (-11.4995, -11.5442) ccw
  arc A817 (2.2419, -11.5442) -> (1.9371, -11.2394) centre (1.9371, -11.5442) ccw
  arc A818 (1.9371, -25.2856) -> (2.2419, -24.9808) centre (1.9371, -24.9808) ccw
  arc A819 (-11.8043, -24.9808) -> (-11.4995, -25.2856) centre (-11.4995, -24.9808) ccw
  line L559 (7.5505, -25.2856) -> (20.9871, -25.2856)
  line L560 (21.2919, -24.9808) -> (21.2919, -11.5442)
  line L561 (20.9871, -11.2394) -> (7.5505, -11.2394)
  line L562 (7.2457, -11.5442) -> (7.2457, -24.9808)
  line L563 (7.2457, -25.2856) -> (21.2919, -11.2394) construction
  line L564 (21.2919, -25.2856) -> (7.2457, -11.2394) construction
  arc A820 (7.5505, -11.2394) -> (7.2457, -11.5442) centre (7.5505, -11.5442) ccw
  arc A821 (21.2919, -11.5442) -> (20.9871, -11.2394) centre (20.9871, -11.5442) ccw
  arc A822 (20.9871, -25.2856) -> (21.2919, -24.9808) centre (20.9871, -24.9808) ccw
  arc A823 (7.2457, -24.9808) -> (7.5505, -25.2856) centre (7.5505, -24.9808) ccw
  line L565 (26.6005, -25.2856) -> (40.0371, -25.2856)
  line L566 (40.3419, -24.9808) -> (40.3419, -11.5442)
  line L567 (40.0371, -11.2394) -> (26.6005, -11.2394)
  line L568 (26.2957, -11.5442) -> (26.2957, -24.9808)
  line L569 (26.2957, -25.2856) -> (40.3419, -11.2394) construction
  line L570 (40.3419, -25.2856) -> (26.2957, -11.2394) construction
  arc A824 (26.6005, -11.2394) -> (26.2957, -11.5442) centre (26.6005, -11.5442) ccw
  arc A825 (40.3419, -11.5442) -> (40.0371, -11.2394) centre (40.0371, -11.5442) ccw
  arc A826 (40.0371, -25.2856) -> (40.3419, -24.9808) centre (40.0371, -24.9808) ccw
  arc A827 (26.2957, -24.9808) -> (26.6005, -25.2856) centre (26.6005, -24.9808) ccw
  line L571 (45.6505, -25.2856) -> (59.0871, -25.2856)
  line L572 (59.3919, -24.9808) -> (59.3919, -11.5442)
  line L573 (59.0871, -11.2394) -> (45.6505, -11.2394)
  line L574 (45.3457, -11.5442) -> (45.3457, -24.9808)
  line L575 (45.3457, -25.2856) -> (59.3919, -11.2394) construction
  line L576 (59.3919, -25.2856) -> (45.3457, -11.2394) construction
  arc A828 (45.6505, -11.2394) -> (45.3457, -11.5442) centre (45.6505, -11.5442) ccw
  arc A829 (59.3919, -11.5442) -> (59.0871, -11.2394) centre (59.0871, -11.5442) ccw
  arc A830 (59.0871, -25.2856) -> (59.3919, -24.9808) centre (59.0871, -24.9808) ccw
  arc A831 (45.3457, -24.9808) -> (45.6505, -25.2856) centre (45.6505, -24.9808) ccw
  line L577 (64.7005, -25.2856) -> (78.1371, -25.2856)
  line L578 (78.4419, -24.9808) -> (78.4419, -11.5442)
  line L579 (78.1371, -11.2394) -> (64.7005, -11.2394)
  line L580 (64.3957, -11.5442) -> (64.3957, -24.9808)
  line L581 (64.3957, -25.2856) -> (78.4419, -11.2394) construction
  line L582 (78.4419, -25.2856) -> (64.3957, -11.2394) construction
  arc A832 (64.7005, -11.2394) -> (64.3957, -11.5442) centre (64.7005, -11.5442) ccw
  arc A833 (78.4419, -11.5442) -> (78.1371, -11.2394) centre (78.1371, -11.5442) ccw
  arc A834 (78.1371, -25.2856) -> (78.4419, -24.9808) centre (78.1371, -24.9808) ccw
  arc A835 (64.3957, -24.9808) -> (64.7005, -25.2856) centre (64.7005, -24.9808) ccw
  line L583 (117.088, -25.2856) -> (130.5246, -25.2856)
  line L584 (130.8294, -24.9808) -> (130.8294, -11.5442)
  line L585 (130.5246, -11.2394) -> (117.088, -11.2394)
  line L586 (116.7832, -11.5442) -> (116.7832, -24.9808)
  line L587 (116.7832, -25.2856) -> (130.8294, -11.2394) construction
  line L588 (130.8294, -25.2856) -> (116.7832, -11.2394) construction
  arc A836 (117.088, -11.2394) -> (116.7832, -11.5442) centre (117.088, -11.5442) ccw
  arc A837 (130.8294, -11.5442) -> (130.5246, -11.2394) centre (130.5246, -11.5442) ccw
  arc A838 (130.5246, -25.2856) -> (130.8294, -24.9808) centre (130.5246, -24.9808) ccw
  arc A839 (116.7832, -24.9808) -> (117.088, -25.2856) centre (117.088, -24.9808) ccw
  line L589 (136.1379, -25.2856) -> (149.5746, -25.2856)
  line L590 (149.8794, -24.9808) -> (149.8794, -11.5442)
  line L591 (149.5746, -11.2394) -> (136.1379, -11.2394)
  line L592 (135.8332, -11.5442) -> (135.8332, -24.9808)
  line L593 (135.8332, -25.2856) -> (149.8794, -11.2394) construction
  line L594 (149.8794, -25.2856) -> (135.8332, -11.2394) construction
  arc A840 (136.1379, -11.2394) -> (135.8332, -11.5442) centre (136.1379, -11.5442) ccw
  arc A841 (149.8794, -11.5442) -> (149.5746, -11.2394) centre (149.5746, -11.5442) ccw
  arc A842 (149.5746, -25.2856) -> (149.8794, -24.9808) centre (149.5746, -24.9808) ccw
  arc A843 (135.8332, -24.9808) -> (136.1379, -25.2856) centre (136.138, -24.9808) ccw
  line L595 (-147.2308, -44.3356) -> (-133.7942, -44.3356)
  line L596 (-133.4894, -44.0308) -> (-133.4894, -30.5942)
  line L597 (-133.7942, -30.2894) -> (-147.2308, -30.2894)
  line L598 (-147.5356, -30.5942) -> (-147.5356, -44.0308)
  line L599 (-147.5356, -44.3356) -> (-133.4894, -30.2894) construction
  line L600 (-133.4894, -44.3356) -> (-147.5356, -30.2894) construction
  arc A844 (-147.2308, -30.2894) -> (-147.5356, -30.5942) centre (-147.2308, -30.5942) ccw
  arc A845 (-133.4894, -30.5942) -> (-133.7942, -30.2894) centre (-133.7942, -30.5942) ccw
  arc A846 (-133.7942, -44.3356) -> (-133.4894, -44.0308) centre (-133.7942, -44.0308) ccw
  arc A847 (-147.5356, -44.0308) -> (-147.2308, -44.3356) centre (-147.2308, -44.0308) ccw
  line L601 (-123.4183, -44.3356) -> (-109.9817, -44.3356)
  line L602 (-109.6769, -44.0308) -> (-109.6769, -30.5942)
  line L603 (-109.9817, -30.2894) -> (-123.4183, -30.2894)
  line L604 (-123.7231, -30.5942) -> (-123.7231, -44.0308)
  line L605 (-123.7231, -44.3356) -> (-109.6769, -30.2894) construction
  line L606 (-109.6769, -44.3356) -> (-123.7231, -30.2894) construction
  arc A848 (-123.4183, -30.2894) -> (-123.7231, -30.5942) centre (-123.4183, -30.5942) ccw
  arc A849 (-109.6769, -30.5942) -> (-109.9817, -30.2894) centre (-109.9817, -30.5942) ccw
  arc A850 (-109.9817, -44.3356) -> (-109.6769, -44.0308) centre (-109.9817, -44.0308) ccw
  arc A851 (-123.7231, -44.0308) -> (-123.4183, -44.3356) centre (-123.4183, -44.0308) ccw
  line L607 (-99.6058, -44.3356) -> (-86.1692, -44.3356)
  line L608 (-85.8644, -44.0308) -> (-85.8644, -30.5942)
  line L609 (-86.1692, -30.2894) -> (-99.6058, -30.2894)
  line L610 (-99.9106, -30.5942) -> (-99.9106, -44.0308)
  line L611 (-99.9106, -44.3356) -> (-85.8644, -30.2894) construction
  line L612 (-85.8644, -44.3356) -> (-99.9106, -30.2894) construction
  arc A852 (-99.6058, -30.2894) -> (-99.9106, -30.5942) centre (-99.6058, -30.5942) ccw
  arc A853 (-85.8644, -30.5942) -> (-86.1692, -30.2894) centre (-86.1692, -30.5942) ccw
  arc A854 (-86.1692, -44.3356) -> (-85.8644, -44.0308) centre (-86.1692, -44.0308) ccw
  arc A855 (-99.9106, -44.0308) -> (-99.6058, -44.3356) centre (-99.6058, -44.0308) ccw
  line L613 (40.888, -44.3356) -> (54.3246, -44.3356)
  line L614 (54.6294, -44.0308) -> (54.6294, -30.5942)
  line L615 (54.3246, -30.2894) -> (40.888, -30.2894)
  line L616 (40.5832, -30.5942) -> (40.5832, -44.0308)
  line L617 (40.5832, -44.3356) -> (54.6294, -30.2894) construction
  line L618 (54.6294, -44.3356) -> (40.5832, -30.2894) construction
  arc A856 (40.888, -30.2894) -> (40.5832, -30.5942) centre (40.888, -30.5942) ccw
  arc A857 (54.6294, -30.5942) -> (54.3246, -30.2894) centre (54.3246, -30.5942) ccw
  arc A858 (54.3246, -44.3356) -> (54.6294, -44.0308) centre (54.3246, -44.0308) ccw
  arc A859 (40.5832, -44.0308) -> (40.888, -44.3356) centre (40.888, -44.0308) ccw
  line L619 (-144.8495, 12.8144) -> (-131.4129, 12.8144)
  line L620 (-131.1081, 13.1192) -> (-131.1081, 26.5558)
  line L621 (-131.4129, 26.8606) -> (-144.8495, 26.8606)
  line L622 (-145.1543, 26.5558) -> (-145.1543, 13.1192)
  line L623 (-145.1543, 12.8144) -> (-131.1081, 26.8606) construction
  line L624 (-131.1081, 12.8144) -> (-145.1543, 26.8606) construction
  arc A860 (-144.8495, 26.8606) -> (-145.1543, 26.5558) centre (-144.8495, 26.5558) ccw
  arc A861 (-131.1081, 26.5558) -> (-131.4129, 26.8606) centre (-131.4129, 26.5558) ccw
  arc A862 (-131.4129, 12.8144) -> (-131.1081, 13.1192) centre (-131.4129, 13.1192) ccw
  arc A863 (-145.1543, 13.1192) -> (-144.8495, 12.8144) centre (-144.8495, 13.1192) ccw
  line L625 (-142.4683, -6.2356) -> (-129.0317, -6.2356)
  line L626 (-128.7269, -5.9308) -> (-128.7269, 7.5058)
  line L627 (-129.0317, 7.8106) -> (-142.4683, 7.8106)
  line L628 (-142.7731, 7.5058) -> (-142.7731, -5.9308)
  line L629 (-142.7731, -6.2356) -> (-128.7269, 7.8106) construction
  line L630 (-128.7269, -6.2356) -> (-142.7731, 7.8106) construction
  arc A864 (-142.4683, 7.8106) -> (-142.7731, 7.5058) centre (-142.4683, 7.5058) ccw
  arc A865 (-128.7269, 7.5058) -> (-129.0317, 7.8106) centre (-129.0317, 7.5058) ccw
  arc A866 (-129.0317, -6.2356) -> (-128.7269, -5.9308) centre (-129.0317, -5.9308) ccw
  arc A867 (-142.7731, -5.9308) -> (-142.4683, -6.2356) centre (-142.4683, -5.9308) ccw
  line L631 (59.938, -44.3356) -> (73.3746, -44.3356)
  line L632 (73.6794, -44.0308) -> (73.6794, -30.5942)
  line L633 (73.3746, -30.2894) -> (59.938, -30.2894)
  line L634 (59.6332, -30.5942) -> (59.6332, -44.0308)
  line L635 (59.6332, -44.3356) -> (73.6794, -30.2894) construction
  line L636 (73.6794, -44.3356) -> (59.6332, -30.2894) construction
  arc A868 (59.938, -30.2894) -> (59.6332, -30.5942) centre (59.938, -30.5942) ccw
  arc A869 (73.6794, -30.5942) -> (73.3746, -30.2894) centre (73.3746, -30.5942) ccw
  arc A870 (73.3746, -44.3356) -> (73.6794, -44.0308) centre (73.3746, -44.0308) ccw
  arc A871 (59.6332, -44.0308) -> (59.938, -44.3356) centre (59.938, -44.0308) ccw
  line L637 (78.988, -44.3356) -> (92.4246, -44.3356)
  line L638 (92.7294, -44.0308) -> (92.7294, -30.5942)
  line L639 (92.4246, -30.2894) -> (78.988, -30.2894)
  line L640 (78.6832, -30.5942) -> (78.6832, -44.0308)
  line L641 (78.6832, -44.3356) -> (92.7294, -30.2894) construction
  line L642 (92.7294, -44.3356) -> (78.6832, -30.2894) construction
  arc A872 (78.988, -30.2894) -> (78.6832, -30.5942) centre (78.988, -30.5942) ccw
  arc A873 (92.7294, -30.5942) -> (92.4246, -30.2894) centre (92.4246, -30.5942) ccw
  arc A874 (92.4246, -44.3356) -> (92.7294, -44.0308) centre (92.4246, -44.0308) ccw
  arc A875 (78.6832, -44.0308) -> (78.988, -44.3356) centre (78.988, -44.0308) ccw
  line L643 (98.038, -44.3356) -> (111.4746, -44.3356)
  line L644 (111.7794, -44.0308) -> (111.7794, -30.5942)
  line L645 (111.4746, -30.2894) -> (98.038, -30.2894)
  line L646 (97.7332, -30.5942) -> (97.7332, -44.0308)